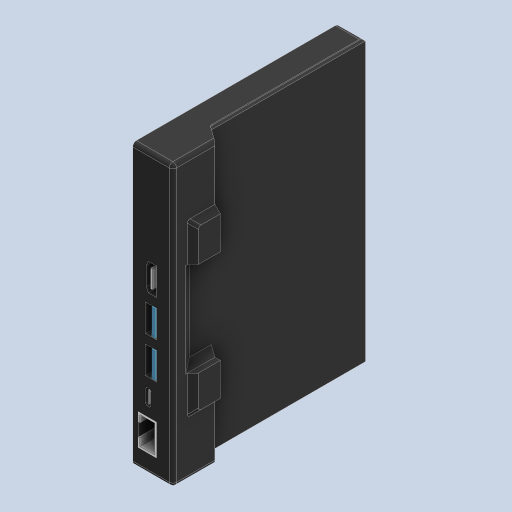
# Autodesk Inventor part: GPD-under
Saved by Autodesk Inventor 2024 (Build 280153000, 153)
## iProperties
Created: 2024-02-10
Part Number: GPD-under
Material: アルミニウム 6061
Document SubType Name: Modeling
Designer: haruy
Density: 2.7 g/cm^3
Appearance: アルミニウム - フラット
Author: haruy
Autodesk Inventor part; units mm, degrees
sketch "スケッチ1" plane through (0, 0, 0) normal (1, 0, 0) x (0, 1, 0)
  line L0 (0, 0) -> (153, 0)
  line L1 (153, 0) -> (153, -113)
  line L2 (153, -113) -> (0, -113)
  line L3 (0, -113) -> (0, 0)
  dimension "d0" = 153
  dimension "d1" = 113
  constraints: 8 end point, 2 parallel, 1 horizontal, 1 perpendicular
  measures "d0" distance of L1.end L2.end
  measures "d1" distance of L0.end L1.end
extrude "押し出し1" add sketch "スケッチ1" along normal blind 22
sketch "スケッチ2" plane through (0, 0, 0) normal (-1, 0, 0) x (0, 0, 1)
  line L0 (-12, 133.5) -> (-18, 133.5)
  line L1 (-18, 133.5) -> (-18, 122.5)
  line L2 (-18, 122.5) -> (-12, 122.5)
  line L3 (-12, 122.5) -> (-12, 133.5)
  line L4 (0, 153) -> (0, 0) projected
  line L5 (-12, 128) -> (-18, 128)
  line L6 (-113, 153) -> (0, 153) projected
  line L7 (0, 76.5) -> (-113, 76.5)
  line L8 (-113, 0) -> (-113, 153) projected
  line L9 (-12, 19.5) -> (-18, 19.5)
  line L10 (-18, 19.5) -> (-18, 30.5)
  line L11 (-18, 30.5) -> (-12, 30.5)
  line L12 (-12, 30.5) -> (-12, 19.5)
  line L13 (-15, 133.5) -> (-15, 122.5)
  line L14 (-113, 153) -> (0, 153) projected
  line L15 (0, 0) -> (-113, 0) projected
  line L16 (-90, 153) -> (-90, 0)
  line L17 (-15, 128) -> (-90, 128)
  line L18 (-52.5, 128) -> (-52.5, 0)
  arc A0 (-12, 133.5) -> (-18, 133.5) centre (-15, 132.25) ccw
  arc A1 (-18, 122.5) -> (-12, 122.5) centre (-15, 123.75) ccw
  arc A2 (-18, 19.5) -> (-12, 19.5) centre (-15, 20.75) ccw
  arc A3 (-12, 30.5) -> (-18, 30.5) centre (-15, 29.25) ccw
  line L19 (-87, 19.5) -> (-87, 30.5)
  line L20 (-93, 30.5) -> (-93, 19.5)
  arc A4 (-93, 19.5) -> (-87, 19.5) centre (-90, 20.75) ccw
  arc A5 (-87, 30.5) -> (-93, 30.5) centre (-90, 29.25) ccw
  arc A6 (-93, 122.5) -> (-87, 122.5) centre (-90, 123.75) ccw
  line L21 (-93, 122.5) -> (-93, 133.5)
  line L22 (-87, 133.5) -> (-87, 122.5)
  arc A7 (-87, 133.5) -> (-93, 133.5) centre (-90, 132.25) ccw
  line L23 (-15, 133.5) -> (-15, 29.25)
  point P0 (-15, 135.5)
  point P1 (-15, 100.5)
  point P2 (-15, 78.5)
  dimension "d4" = 6
  dimension "d5" = 11
  dimension "d6" = 12
  dimension "d7" = 25
  dimension "d8" = 75
  dimension "d10" = 2
  dimension "d14" = 35
  dimension "d15" = 22
  constraints: 38 end point, 19 symmetric about line, 17 point on circle, 8 centre point, 8 midpoint, 6 point on line, 4 perpendicular, 3 parallel, 1 horizontal, 7 other
  measures "d4" distance of L2.end L1.end
  measures "d5" distance of L1.end L0.end
  measures "d6" distance between parallel lines of L3 L4
  measures "d7" distance between parallel lines of L6 L5
  measures "d8" distance between parallel lines of L16 L13
  measures "d10" distance from line of point (-15, 135.5) L0
  measures "d14" distance of point (-15, 135.5) point (-15, 100.5)
  measures "d15" distance of point (-15, 100.5) point (-15, 78.5)
extrude "押し出し2" add sketch "スケッチ2" along normal blind 3 separate body contours L3 L5 L13 L0 | L0 A0 | L13 L5 L1 L0 | L3 L2 L13 L5 | L13 L2 L1 L5 | A1 L23 L2 | L23 A1 L2 | L22 A6 L16 L17 | L17 L16 A7 L22 | L16 A6 L21 A7 | A5 L19 A4 L16 | L16 A4 L20 A5 | A2 L9 | L9 L10 L11 L12 | L11 L23 A3 | A3 L23 L11
fillet "フィレット1" radius 2 16 edges at (-3, 128, -93) (-3, 128, -87) (-3, 120.5, -90) (-3, 135.5, -90) (-3, 25, -93) (-3, 32.5, -90) (-3, 17.5, -90) (-3, 25, -87) (-3, 25, -12) (-3, 17.5, -15) (-3, 25, -18) (-3, 32.5, -15) (-3, 128, -18) (-3, 120.5, -15) (-3, 135.5, -15) (-3, 128, -12)
hole "穴1" at (0, 100.5, -15) at (0, 78.5, -15) direction (1, 0, 0) diameter 3 depth 5 bodies 1
thread "ねじ1" size "M3x0.5" class "6H" standard "ANSI Metric M Profile" full length
thread "ねじ2" size "M3x0.5" class "6H" standard "ANSI Metric M Profile" full length
sketch "スケッチ4" plane through (0, 0, -113) normal (0, -1, 0) x (1, 0, 0)
  line L0 (0, 0) -> (22, 0) projected
  line L1 (15, 0) -> (15, 85)
  line L2 (15, 85) -> (22, 90)
  line L3 (22, 0) -> (22, 113) projected
  line L4 (15, 85) -> (22, 85)
  line L5 (13, 0) -> (13, 82.5422)
  line L6 (15, 85) -> (13.8375, 84.1697)
  arc A0 (13.8375, 84.1697) -> (13, 82.5422) centre (15, 82.5422) ccw
  line L7 (11, 85) -> (5, 85)
  line L8 (5, 85) -> (5, 70)
  line L9 (5, 70) -> (11, 70)
  line L10 (11, 70) -> (11, 85)
  line L11 (0, 113) -> (0, 0) projected
  line L12 (11, 70) -> (8, 70)
  line L13 (8, 70) -> (8, 85)
  line L14 (8, 85) -> (11, 85)
  line L15 (11, 85) -> (11, 70)
  line L16 (10.5, 70.5) -> (8.5, 70.5)
  line L17 (8.5, 70.5) -> (8.5, 84.5)
  line L18 (8.5, 84.5) -> (10.5, 84.5)
  line L19 (10.5, 84.5) -> (10.5, 70.5)
  line L20 (9, 66) -> (7, 66)
  line L21 (7, 66) -> (7, 54)
  line L22 (7, 54) -> (9, 54)
  line L23 (9, 54) -> (9, 66)
  point P0 (13, 83.5714)
  point P1 (13, 83.5714)
  dimension "d27" = 85
  dimension "d28" = 5
  dimension "d29" = 7
  dimension "d30" = 2
  dimension "d31" = 0
  dimension "d32" = 2
  dimension "d54" = 6
  dimension "d55" = 15
  dimension "d56" = 70
  dimension "d57" = 5
  dimension "d60" = 3
  dimension "d61" = 15
  dimension "d64" = 0.5
  dimension "d67" = 2
  dimension "d68" = 12
  dimension "d69" = 4
  dimension "d70" = 1
  constraints: 42 end point, 8 parallel, 6 point on line, 4 horizontal, 4 perpendicular, 2 point on circle, 2 tangent, 2 vertical, 1 centre point, 3 other
  measures "d27" distance of L1.start L1.end
  measures "d28" distance of L2.end L4.end
  measures "d29" distance between parallel lines of L1 L3
  measures "d30" distance between parallel lines of L5 L1
  measures "d31" distance of point (13, 83.571) point (13, 83.571)
  measures "d32" radius of A0
  measures "d54" distance of L9.end L8.end
  measures "d55" distance of L8.end L7.end
  measures "d56" distance between parallel lines of L0 L9
  measures "d57" distance between parallel lines of L11 L8
  measures "d60" distance of L13.end L14.end
  measures "d61" distance of L12.end L13.end
  measures "d64" distance between parallel lines of L15 L19
  measures "d67" distance of L22.end L21.end
  measures "d68" distance of L21.end L20.end
  measures "d69" distance between parallel lines of L12 L20
  measures "d70" distance between parallel lines of L13 L23
extrude "押し出し3" cut sketch "スケッチ4" against normal blind 0.5 contours L5 A0 L6 L1 L0 bodies 1
extrude "押し出し4" cut sketch "スケッチ4" against normal through all contours L1 L4 L3 L0 | L2 L3 L4 bodies 1
sketch "スケッチ5" plane through (0, 0, -113) normal (0, 0, -1) x (-1, 0, 0)
  line L0 (0, 0) -> (-13, 0) projected
  line L1 (-13, 0) -> (-13, 153)
  line L2 (0, 153) -> (-15, 153) projected
  line L3 (-15, 0.5) -> (-13, 0.5)
  line L4 (-13, 0.5) -> (-13, 153)
  line L5 (-13, 153) -> (-15, 153)
  line L6 (-15, 153) -> (-15, 0.5)
  constraints: 10 end point, 2 parallel, 1 horizontal, 1 perpendicular, 1 point on line, 1 vertical
extrude "押し出し5" cut sketch "スケッチ5" against normal blind 0.5 bodies 1
sketch "スケッチ6" plane through (0, 153, 0) normal (0, 1, 0) x (1, 0, 0)
  line L0 (13, 112.5) -> (13, 113) projected
  line L1 (22, 23) -> (15, 28) projected
  line L2 (13, 112.5) -> (15, 112.5)
  line L3 (15, 112.5) -> (15, 28)
  line L4 (15, 28) -> (13, 28)
  line L5 (13, 30.4578) -> (13, 112.5)
  line L6 (15, 28) -> (13.8375, 28.8303)
  arc A0 (13, 30.4578) -> (13.8375, 28.8303) centre (15, 30.4578) ccw
  point P0 (0, 0)
  dimension "d39" = 2
  constraints: 10 end point, 2 parallel, 2 point on circle, 2 tangent, 1 centre point, 1 horizontal, 1 perpendicular, 1 point on line
  measures "d39" radius of A0
extrude "押し出し6" cut sketch "スケッチ6" against normal blind 0.5 bodies 1
sketch "スケッチ7" plane through (0, 0, -113) normal (0, 0, -1) x (-1, 0, 0)
  line L0 (0, 0) -> (-13, 0) projected
  line L1 (-13, 153) -> (-13, 0) projected
  circle A0 centre (-7.5, 17.5) radius 4.5
  dimension "d42" = 17.5
  dimension "d43" = 5.5
  dimension "d51" = 9
  constraints: 1 centre point, 1 coincident
  measures "d42" distance from line of L0 point (-7.5, 17.5)
  measures "d43" distance from line of point (-7.5, 17.5) L1
  measures "d51" diameter of A0
hole "穴2" at (7.5, 17.5, -113) direction (0, 0, 1) diameter 4 depth 5 bodies 1
extrude "押し出し7" cut sketch "スケッチ7" against normal blind 0.5 bodies 1
extrude "押し出し8" cut sketch "スケッチ4" against normal blind 10 contours L10 L9 L13 L7 | L13 L9 L8 L7 | L16 L17 L18 L19 bodies 1
extrude "押し出し10" add sketch "スケッチ4" against normal blind 10 separate body contours L16 L17 L18 L19
extrude "押し出し11" cut sketch "スケッチ4" against normal blind 10 contours L23 L22 L21 L20 bodies 1
sketch "スケッチ9" plane through (0, 0, 0) normal (0, 0, 1) x (1, 0, 0)
  line L0 (13, 27) -> (3, 27)
  line L1 (3, 27) -> (3, 10)
  line L2 (3, 10) -> (13, 10)
  line L3 (13, 10) -> (13, 27)
  line L4 (0, 153) -> (0, 0) projected
  line L5 (0, 0) -> (22, 0) projected
  line L6 (12, 26) -> (4, 26)
  line L7 (4, 26) -> (4, 11)
  line L8 (4, 11) -> (12, 11)
  line L9 (12, 11) -> (12, 26)
  line L10 (4, 22) -> (3, 22)
  line L11 (4, 15) -> (3, 15)
  line L12 (10, 40) -> (7, 40)
  line L13 (7, 40) -> (7, 33)
  line L14 (7, 33) -> (10, 33)
  line L15 (10, 33) -> (10, 40)
  arc A0 (10, 40) -> (7, 40) centre (8.5, 39.375) ccw
  line L16 (10, 36.5) -> (7, 36.5)
  arc A1 (7, 33) -> (10, 33) centre (8.5, 33.625) ccw
  line L17 (8.75, 40) -> (8.25, 40)
  line L18 (8.25, 40) -> (8.25, 33)
  line L19 (8.25, 33) -> (8.75, 33)
  line L20 (8.75, 33) -> (8.75, 40)
  line L21 (13, 61) -> (7, 61)
  line L22 (7, 61) -> (7, 46)
  line L23 (7, 46) -> (13, 46)
  line L24 (13, 46) -> (13, 61)
  line L25 (10, 61) -> (10, 46)
  line L26 (13, 61) -> (10, 61)
  line L27 (10, 61) -> (10, 46)
  line L28 (10, 46) -> (13, 46)
  line L29 (13, 46) -> (13, 61)
  line L30 (10, 46.5) -> (12.5, 46.5)
  line L31 (12.5, 46.5) -> (12.5, 61)
  line L32 (13, 60.5) -> (10.5, 60.5)
  line L33 (10.5, 60.5) -> (10.5, 46)
  line L34 (7, 81) -> (13, 81)
  line L35 (13, 81) -> (13, 66)
  line L36 (13, 66) -> (7, 66)
  line L37 (7, 66) -> (7, 81)
  line L38 (13, 81) -> (10, 81)
  line L39 (10, 81) -> (10, 66)
  line L40 (10, 66) -> (13, 66)
  line L41 (13, 66) -> (13, 81)
  line L42 (10.5, 66.5) -> (10.5, 80.5)
  line L43 (10.5, 80.5) -> (12.5, 80.5)
  line L44 (12.5, 80.5) -> (12.5, 66.5)
  line L45 (12.5, 66.5) -> (10.5, 66.5)
  line L46 (13, 101) -> (8.5, 101)
  line L47 (8.5, 101) -> (8.5, 86)
  line L48 (8.5, 86) -> (13, 86)
  line L49 (13, 86) -> (13, 101)
  line L50 (7.5, 98.5) -> (7.5, 88.5)
  line L51 (8.5, 101) -> (7.5, 98.5)
  line L52 (7.5, 88.5) -> (8.5, 86)
  line L53 (9.75, 98.5) -> (10.75, 98.5)
  line L54 (10.75, 98.5) -> (10.75, 88.5)
  line L55 (10.75, 88.5) -> (9.75, 88.5)
  line L56 (9.75, 88.5) -> (9.75, 98.5)
  point P0 (8.5, 41)
  point P1 (10.5, 46.5)
  point P2 (12.5, 60.5)
  point P3 (9.75, 93.5)
  dimension "d73" = 10
  dimension "d74" = 17
  dimension "d75" = 3
  dimension "d76" = 10
  dimension "d77" = 1
  dimension "d78" = 5
  dimension "d79" = 5
  dimension "d84" = 3
  dimension "d85" = 7
  dimension "d86" = 7
  dimension "d87" = 6
  dimension "d88" = 1
  dimension "d89" = 0.5
  dimension "d90" = 0.25
  dimension "d95" = 6
  dimension "d96" = 15
  dimension "d97" = 7
  dimension "d98" = 5
  dimension "d99" = 0.5
  dimension "d100" = 0.5
  dimension "d105" = 6
  dimension "d106" = 15
  dimension "d107" = 5
  dimension "d108" = 0
  dimension "d109" = 3
  dimension "d110" = 15
  dimension "d111" = 0.5
  dimension "d116" = 4.5
  dimension "d117" = 15
  dimension "d118" = 0
  dimension "d119" = 5
  dimension "d120" = 10
  dimension "d121" = 1
  dimension "d122" = 2.5
  dimension "d123" = 1
  dimension "d124" = 10
  dimension "d126" = 2.5
  dimension "d128" = 2.25
  constraints: 110 end point, 22 parallel, 14 perpendicular, 9 horizontal, 6 point on line, 5 midpoint, 5 point on circle, 2 centre point, 1 symmetric about line, 1 vertical, 9 other
  measures "d73" distance of L2.end L1.end
  measures "d74" distance of L1.end L0.end
  measures "d75" distance between parallel lines of L4 L1
  measures "d76" distance between parallel lines of L5 L2
  measures "d77" distance between parallel lines of L3 L9
  measures "d78" distance between parallel lines of L0 L10
  measures "d79" distance between parallel lines of L11 L2
  measures "d84" distance of L14.end L13.end
  measures "d85" distance of L13.end L12.end
  measures "d86" distance between parallel lines of L13 L4
  measures "d87" distance between parallel lines of L14 L0
  measures "d88" distance from line of point (8.5, 41) L12
  measures "d89" distance of L19.end L18.end
  measures "d90" distance from line of A0.centre L20
  measures "d95" distance of L23.end L22.end
  measures "d96" distance of L22.end L21.end
  measures "d97" distance between parallel lines of L4 L22
  measures "d98" distance from line of L23 point (8.5, 41)
  measures "d99" distance between parallel lines of L28 L30
  measures "d100" distance between parallel lines of L26 L32
  measures "d105" distance of L35.end L36.end
  measures "d106" distance of L34.end L35.end
  measures "d107" distance between parallel lines of L36 L21
  measures "d108" distance between parallel lines of L37 L22
  measures "d109" distance of L40.end L39.end
  measures "d110" distance of L39.end L38.end
  measures "d111" distance between parallel lines of L39 L42
  measures "d116" distance of L48.end L47.end
  measures "d117" distance of L47.end L46.end
  measures "d118" distance between parallel lines of L49 L35
  measures "d119" distance between parallel lines of L48 L34
  measures "d120" distance of L50.start L50.end
  measures "d121" distance between parallel lines of L50 L47
  measures "d122" vertical distance of L50.start L46.end
  measures "d123" distance of L54.end L55.end
  measures "d124" distance of L53.end L54.end
  measures "d126" distance between parallel lines of L46 L53
  measures "d128" distance between parallel lines of L50 L56
extrude "押し出し12" cut sketch "スケッチ9" against normal blind 10 contours L3 L2 L1 L11 L7 L8 L9 L6 L10 L0 | L10 L7 L11 L1 | L7 L6 L9 L8 bodies 1
extrude "押し出し13" add sketch "スケッチ9" against normal blind 10 separate body contours L3 L2 L1 L11 L7 L8 L9 L6 L10 L0
extrude "押し出し14" cut sketch "スケッチ9" against normal blind 10 contours L15 L16 L20 L12 | L12 A0 | L20 L16 L18 L12 | L15 L14 L20 L16 | L12 L18 L16 L13 | L20 L14 L18 L16 | A1 L14 | L16 L18 L14 L13 bodies 1
extrude "押し出し15" add sketch "スケッチ9" against normal blind 10 separate body contours L20 L16 L18 L12 | L20 L14 L18 L16
extrude "押し出し16" cut sketch "スケッチ9" against normal blind 10 contours L24 L32 L31 L21 | L31 L32 L33 L30 L25 L21 | L24 L23 L33 L30 L31 L32 | L25 L23 L22 L21 | L31 L30 L33 L32 | L30 L33 L23 L25 bodies 1
extrude "押し出し17" add sketch "スケッチ9" against normal blind 10 separate body contours L31 L30 L33 L32
extrude "押し出し18" cut sketch "スケッチ9" against normal blind 10 contours L34 L39 L36 L37 | L34 L35 L36 L39 | L42 L43 L44 L45 bodies 1
extrude "押し出し19" add sketch "スケッチ9" against normal blind 10 separate body contours L42 L43 L44 L45
extrude "押し出し20" cut sketch "スケッチ9" against normal blind 10 contours L49 L48 L47 L46 | L47 L52 L50 L51 | L53 L54 L55 L56 bodies 1
extrude "押し出し21" add sketch "スケッチ9" against normal blind 10 separate body contours L53 L54 L55 L56
sketch "スケッチ11" plane through (22, 0, 0) normal (1, 0, 0) x (0, 0, -1)
  line L0 (0, 153) -> (0, 0) projected
  line L1 (0, 76.5) -> (23, 76.5)
  line L2 (23, 0) -> (23, 153) projected
  line L3 (7.0744, 50.75) -> (16.5, 50.75)
  line L4 (16.5, 50.75) -> (16.5, 102.25)
  line L5 (16.5, 102.25) -> (7.0744, 102.25)
  line L6 (7.0744, 102.25) -> (7.0744, 50.75)
  line L7 (16.5, 50.75) -> (23, 50.75)
  line L8 (16.5, 102.25) -> (23, 102.25)
  line L9 (23, 50.75) -> (11, 50.75)
  line L10 (11, 50.75) -> (11, 32.75)
  line L11 (11, 32.75) -> (23, 32.75)
  line L12 (23, 32.75) -> (23, 50.75)
  line L13 (23, 102.25) -> (11, 102.25)
  line L14 (11, 102.25) -> (11, 120.25)
  line L15 (11, 120.25) -> (23, 120.25)
  line L16 (23, 120.25) -> (23, 102.25)
  line L17 (8, 29.75) -> (8, 53.75)
  line L18 (8, 123.25) -> (8, 99.25)
  line L19 (8, 99.25) -> (26, 99.25)
  line L20 (26, 99.25) -> (26, 123.25)
  line L21 (26, 123.25) -> (8, 123.25)
  line L22 (8, 29.75) -> (23, 29.75)
  line L23 (23, 29.75) -> (23, 50.75)
  line L24 (23, 50.75) -> (8, 50.75)
  line L25 (8, 50.75) -> (8, 29.75)
  line L26 (28, 0) -> (28, 10) projected
  line L27 (28, 0.5) -> (28, 152.5) projected
  line L28 (28, 0) -> (28, 152.5)
  dimension "d133" = 51.5
  dimension "d134" = 25.75
  dimension "d135" = 12
  dimension "d136" = 18
  dimension "d137" = 12
  dimension "d138" = 18
  dimension "d143" = 3
  dimension "d144" = 3
  dimension "d153" = 3
  constraints: 50 end point, 10 parallel, 7 perpendicular, 4 horizontal, 2 midpoint, 2 point on line, 1 vertical, 3 other
  measures "d133" distance of L4.end L3.end
  measures "d134" distance between parallel lines of L3 L1
  measures "d135" distance of L11.end L10.end
  measures "d136" distance of L10.end L9.end
  measures "d137" distance of L14.end L15.end
  measures "d138" distance of L13.end L14.end
  measures "d143" distance between parallel lines of L10 L17
  measures "d144" distance between parallel lines of L14 L18
  measures "d153" distance between parallel lines of L22 L11
ref_plane "作業平面1" through (0, 76.5, 0) normal (0, 1, 0) x (1, 0, 0)
ref_plane "作業平面2" through (25, 0, 0) normal (1, 0, 0) x (0, 0, -1)
sketch "スケッチ15" plane through (25, 0, 0) normal (1, 0, 0) x (0, 0, -1)
  line L0 (11, 32.75) -> (23, 32.75)
  line L1 (23, 32.75) -> (23, 50.75)
  line L2 (23, 50.75) -> (11, 50.75)
  line L3 (11, 50.75) -> (11, 32.75)
  line L4 (0, 153) -> (0, 0) projected
  line L5 (0, 0) -> (23, 0) projected
  dimension "d166" = 12
  dimension "d167" = 18
  dimension "d168" = 11
  dimension "d169" = 32.75
  constraints: 8 end point, 2 parallel, 1 horizontal, 1 perpendicular
  measures "d166" distance of L2.end L1.end
  measures "d167" distance of L1.end L0.end
  measures "d168" distance between parallel lines of L3 L4
  measures "d169" distance between parallel lines of L5 L0
loft "ロフト2" add profiles "スケッチ15", "スケッチ11" separate body contours all / L7 L2 L11 L10 L3 | L3 L10 L11 L2 L22 L17
mirror "ミラー2" about plane through (0, 76.5, 0) normal (0, 1, 0) of "ロフト2" bodies 9
fillet "フィレット6" radius 2 2 edges at (23.5, 31.25, -9.5) (23.5, 121.75, -9.5)
fillet "フィレット7" radius 2 3 edges at (22, 153, -11.5) (22, 76.5, 0) (22, 0, -11.5)
fillet "フィレット8" radius 2 6 edges at (6.5, 0, -113) (6.5, 153, -113) (21.4142, 0.5858, -0.5858) (10, 0, 0) (21.4142, 152.4142, -0.5858) (10, 153, 0)
sketch "スケッチ16" plane through (22, 50.75, -23) normal (0, 1, 0) x (1, 0, 0)
  line L0 (0, 0) -> (0, -15) projected
  line L1 (0, -15) -> (-7, -15)
  line L2 (-7, -15) -> (-7, 5)
  line L3 (-7, 5) -> (0, 5)
  line L4 (0, 5) -> (0, -15)
  line L5 (-7, -7.0183) -> (0, -16)
  line L6 (0, -16) -> (0, -15)
  line L7 (0, 0) -> (-7, 5)
  line L8 (0, -16) -> (-7, -16)
  line L9 (-7, -16) -> (-7, -15)
  point P0 (-22, -23)
  dimension "d177" = 7
  dimension "d178" = 20
  dimension "d181" = 21
  constraints: 18 end point, 2 horizontal, 2 parallel, 2 perpendicular, 1 point on line, 1 vertical
  measures "d177" distance of L2.end L3.end
  measures "d178" distance of L1.end L2.end
  measures "d181" distance of L3.end L5.end
ref_plane "作業平面3" through (0, 2, -28) normal (0, 0, 1) x (1, 0, 0)
sketch "スケッチ17" plane through (0, 2, -28) normal (0, 0, 1) x (1, 0, 0)
  line L0 (15, -1.5) -> (15, 150.5) projected
  line L1 (15, 48.75) -> (25.7773, 48.75)
  line L2 (25.7773, 48.75) -> (25.7773, 100.25)
  line L3 (25.7773, 100.25) -> (15, 100.25)
  line L4 (15, 100.25) -> (15, 48.75)
  point P0 (0, -2)
  point P1 (13, -2)
  dimension "d183" = 51.5
  dimension "d185" = 50.75
  constraints: 8 end point, 2 parallel, 1 horizontal, 1 perpendicular, 1 point on line
  measures "d183" distance of L2.end L1.end
  measures "d185" distance from line of L1 point (13, -2)
extrude "押し出し27" cut sketch "スケッチ17" along normal blind 21 bodies 1
extrude "押し出し28" add sketch "スケッチ16" along normal up to surface (51.5 mm away) contours L5 L8 L9 L1 | L1 L2 L5 bodies 9
equation "\"d126\" = d122"
